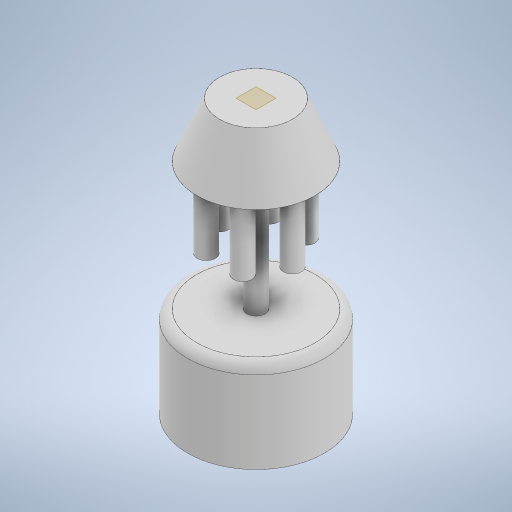
# Autodesk Inventor part: Main_Tower
Saved by Autodesk Inventor 2024.3 (Build 283343000, 343)
## iProperties
Created: 2024-08-06
Part Number: Main_Tower
Material: Generic
Document SubType Name: Modeling
Designer: lordk
Density: 1 g/cm^3
Appearance: Default
Author: lordk
Autodesk Inventor part; units mm, degrees
ref_plane "YZ Plane" through (0, 0, 0) normal (1, 0, 0) x (0, 1, 0)
ref_plane "XZ Plane" through (0, 0, 0) normal (0, 1, 0) x (-1, 0, 0)
ref_plane "XY Plane" through (0, 0, 0) normal (0, 0, 1) x (1, 0, 0)
sketch "Sketch1" plane through (0, 0, 0) normal (0, 1, 0) x (-1, 0, 0)
  circle A0 centre (0, 0) radius 37.5
  dimension "d0" = 75
  constraints: 1 centre point, 1 coincident
  measures "d0" diameter of A0
extrude "Extrusion1" add sketch "Sketch1" along normal blind 50
fillet "Fillet1" radius 5 1 edges at (37.5, 50, 0)
sketch "Sketch2" plane through (0, 50, 0) normal (0, 1, 0) x (1, 0, 0)
  circle A0 centre (0, 0) radius 5
  dimension "d4" = 10
  constraints: 1 centre point, 1 coincident
  measures "d4" diameter of A0
extrude "Extrusion2" add sketch "Sketch2" along normal blind 70
sketch "Sketch3" plane through (0, 120, 0) normal (0, 1, 0) x (1, 0, 0)
  circle A0 centre (0, 0) radius 32.5
  dimension "d7" = 65
  constraints: 1 centre point, 1 coincident
  measures "d7" diameter of A0
ref_plane "Work Plane1" through (0, 150, 0) normal (0, 1, 0) x (1, 0, 0)
sketch "Sketch4" plane through (0, 150, 0) normal (0, 1, 0) x (1, 0, 0)
  circle A0 centre (0, 0) radius 20
  dimension "d9" = 40
  constraints: 1 centre point, 1 coincident
  measures "d9" diameter of A0
loft "Loft1" add profiles "Sketch3", "Sketch4"
sketch "Sketch5" plane through (0, 120, 0) normal (0, -1, 0) x (1, 0, 0)
  circle A0 centre (0, 0) radius 20 projected
  circle A1 centre (-20, 0) radius 5
  circle A2 centre (0, 0) radius 5 projected
  circle A3 centre (-10, -17.3205) radius 5
  circle A4 centre (10, -17.3205) radius 5
  circle A5 centre (20, 0) radius 5
  circle A6 centre (10, 17.3205) radius 5
  circle A7 centre (-10, 17.3205) radius 5
  dimension "d14" = 10
  dimension "d15" = 20
  dimension "d18" = 360
  constraints: 6 centre point, 1 horizontal alignment, 14 other
  measures "d14" diameter of A1
  measures "d15" distance of A2.centre A1.centre
extrude "Extrusion3" add sketch "Sketch5" along normal blind 40 contours A0 A5 | A0 A5 | A6 A0 | A0 A6 | A4 A0 | A0 A4 | A7 A0 | A0 A7 | A3 A0 | A0 A3 | A1 A0 | A0 A1
body "Solid1"
